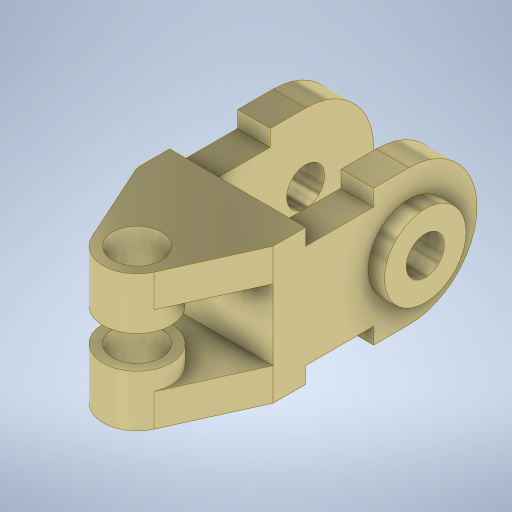
# Autodesk Inventor part: Opakování_1
Saved by Autodesk Inventor 2023 (Build 270158000, 158)
## iProperties
Created: 2023-11-21
Part Number: Opakování_1
Material: Stříbro
Document SubType Name: Modeling
Designer: bit40248
Density: 10.49 g/cm^3
Appearance: Zlato – kov
Mass: 1272.72 g
Surface Area: 310.869 cm^2
Volume: 121.327 cm^3
Author: bit40248
Autodesk Inventor part; units mm, degrees
ref_plane "YZ Plane" through (0, 0, 0) normal (1, 0, 0) x (0, 1, 0)
ref_plane "XZ Plane" through (0, 0, 0) normal (0, 1, 0) x (-1, 0, 0)
ref_plane "XY Plane" through (0, 0, 0) normal (0, 0, 1) x (1, 0, 0)
sketch "Náčrt1" plane through (0, 0, 0) normal (0, 0, 1) x (1, 0, 0)
  line L0 (0, 0) -> (50, 0)
  line L1 (50, 0) -> (50, -50)
  line L2 (50, -50) -> (0, -50)
  line L3 (0, -50) -> (0, 0)
  dimension "d0" = 50
  dimension "d1" = 50
  constraints: 8 end point, 2 parallel, 1 horizontal, 1 perpendicular
  measures "d0" distance of L1.end L2.end
  measures "d1" distance of L0.end L1.end
extrude "Vysunutí1" add sketch "Náčrt1" against normal blind 50
sketch "Náčrt2" plane through (0, 0, 0) normal (0, 1, 0) x (1, 0, 0)
  line L0 (12, 12) -> (38, 12)
  line L1 (38, 12) -> (38, 50)
  line L2 (38, 50) -> (12, 50)
  line L3 (12, 50) -> (12, 12)
  line L4 (0, 50) -> (50, 50) projected
  line L5 (0, 0) -> (0, 50) projected
  dimension "d4" = 12
  dimension "d5" = 26
  dimension "d6" = 38
  constraints: 8 end point, 2 parallel, 1 collinear, 1 horizontal, 1 perpendicular
  measures "d4" distance between parallel lines of L5 L3
  measures "d5" distance between parallel lines of L1 L3
  measures "d6" distance between parallel lines of L0 L2
extrude "Vysunutí2" cut sketch "Náčrt2" against normal blind 50
sketch "Náčrt3" plane through (50, -50, 0) normal (1, 0, 0) x (0, 0, -1)
  line L0 (12, 50) -> (37, 50)
  line L1 (37, 50) -> (37, 44)
  line L2 (37, 44) -> (12, 44)
  line L3 (12, 44) -> (12, 50)
  line L4 (0, 50) -> (50, 50) projected
  line L5 (0, 0) -> (0, 50) projected
  point P0 (37, 47)
  point P1 (12, 47)
  dimension "d9" = 12
  dimension "d10" = 25
  dimension "d11" = 6
  constraints: 8 end point, 2 midpoint, 2 parallel, 1 collinear, 1 horizontal, 1 perpendicular
  measures "d9" distance between parallel lines of L5 L3
  measures "d10" distance of point (37, 47) point (12, 47)
  measures "d11" distance between parallel lines of L2 L4
extrude "Vysunutí3" cut sketch "Náčrt3" against normal blind 50
sketch "Náčrt4" plane through (50, -50, 0) normal (1, 0, 0) x (0, 0, -1)
  line L0 (12, 6) -> (37, 6)
  line L1 (37, 6) -> (37, 0)
  line L2 (37, 0) -> (12, 0)
  line L3 (12, 0) -> (12, 6)
  line L4 (0, 0) -> (50, 0) projected
  line L5 (0, 0) -> (0, 50) projected
  point P0 (37, 3)
  point P1 (12, 3)
  dimension "d14" = 12
  dimension "d15" = 6
  dimension "d16" = 25
  constraints: 8 end point, 2 midpoint, 2 parallel, 1 collinear, 1 horizontal, 1 perpendicular
  measures "d14" distance between parallel lines of L5 L3
  measures "d15" distance between parallel lines of L2 L0
  measures "d16" distance of point (37, 3) point (12, 3)
extrude "Vysunutí4" cut sketch "Náčrt4" against normal blind 50
sketch "Náčrt5" plane through (50, -50, 0) normal (1, 0, 0) x (0, 0, -1)
  line L0 (50, 0) -> (50, 50) projected
  arc A0 (50, 0) -> (50, 50) centre (50, 25) ccw
  point P0 (0, 50)
  constraints: 2 end point, 2 point on circle, 1 centre point, 1 midpoint
extrude "Vysunutí5" add sketch "Náčrt5" against normal blind 50
sketch "Náčrt6" plane through (38, 0, -37) normal (0, 1, 0) x (1, 0, 0)
  line L0 (-26, 13) -> (-38, 13) projected
  line L1 (-26, 13) -> (0, 13)
  line L2 (0, 13) -> (0, 55.1409)
  line L3 (0, 55.1409) -> (-26, 55.1409)
  line L4 (-26, 55.1409) -> (-26, 13)
  point P0 (-38, -37)
  constraints: 8 end point, 2 parallel, 1 horizontal, 1 perpendicular
extrude "Vysunutí6" cut sketch "Náčrt6" against normal blind 50
sketch "Náčrt7" plane through (50, -50, 0) normal (1, 0, 0) x (0, 0, -1)
  circle A0 centre (50, 25) radius 15
  point P0 (0, 50)
  dimension "d23" = 30
  constraints: 1 centre point
  measures "d23" diameter of A0
extrude "Vysunutí7" add sketch "Náčrt7" along normal blind 6
sketch "Náčrt8" plane through (0, -50, 0) normal (-1, 0, 0) x (0, 0, 1)
  circle A0 centre (-50, 25) radius 15 projected
  circle A1 centre (-50, 25) radius 15
  point P0 (0, 50)
  constraints: 1 centre point, 1 coincident
extrude "Vysunutí8" add sketch "Náčrt8" along normal blind 6
sketch "Náčrt9" plane through (-6, -25, -50) normal (-1, 0, 0) x (0, 0, 1)
  circle A0 centre (0, 0) radius 7
  point P0 (50, 25)
  dimension "d28" = 14
  constraints: 1 centre point
  measures "d28" diameter of A0
extrude "Vysunutí9" cut sketch "Náčrt9" against normal blind 100
sketch "Náčrt10" plane through (0, 0, 0) normal (0, 1, 0) x (1, 0, 0)
  circle A0 centre (25, -25) radius 12.5
  line L0 (0, 0) -> (13.607, -30.143)
  line L1 (50, 0) -> (50, 12) projected
  line L2 (50, 0) -> (36.393, -30.143)
  dimension "d31" = 25
  constraints: 4 end point, 2 point on circle, 2 tangent, 1 centre point, 1 other
  measures "d31" diameter of A0
extrude "Vysunutí10" add sketch "Náčrt10" against normal blind 50
sketch "Náčrt11" plane through (25, 0, 25) normal (0, 1, 0) x (1, 0, 0)
  point P0 (-25, 25)
sketch "Náčrt12" plane through (0, 0, 0) normal (0, 1, 0) x (1, 0, 0)
  line L0 (50, 0) -> (0, 0) projected
  line L1 (0, 0) -> (13.607, -30.143)
  line L2 (50, 0) -> (36.393, -30.143)
  circle A0 centre (25, -25) radius 12.5 projected
  constraints: 4 end point, 2 point on circle, 2 tangent
extrude "Vysunutí11" add sketch "Náčrt12" against normal blind 12 contours L2 A0 L1 L0
sketch "Náčrt13" plane through (0, -50, 0) normal (0, -1, 0) x (1, 0, 0)
  line L0 (50, 0) -> (50, -12) projected
  line L1 (50, 0) -> (36.393, 30.143)
  line L2 (13.607, 30.143) -> (0, 0) projected
  line L3 (0, 0) -> (13.607, 30.143)
  circle A0 centre (25, 25) radius 12.5 projected
  line L4 (50, 0) -> (50, -12) projected
  line L5 (0, 0) -> (0, -12) projected
  line L6 (50, 0) -> (0, 0)
  constraints: 6 end point, 2 point on circle, 2 tangent
extrude "Vysunutí12" add sketch "Náčrt13" against normal blind 12 contours L6 L2 A0 L1
sketch "Náčrt16" plane through (0, 0, 0) normal (0, 0, 1) x (1, 0, 0)
  point P0 (0, 0)
sketch "Náčrt17" plane through (0, 0, 0) normal (0, 0, 1) x (1, 0, 0)
  point P0 (0, 0)
sketch "Náčrt18" plane through (0, 0, 0) normal (0, 0, 1) x (1, 0, 0)
  line L0 (50, -10) -> (50, -40) projected
  line L1 (0, 0) -> (0, -50) projected
  line L2 (50, -19) -> (0, -19)
  line L3 (0, -19) -> (0, -31)
  line L4 (0, -31) -> (50, -31)
  line L5 (50, -31) -> (50, -19)
  dimension "d38" = 12
  constraints: 8 end point, 2 parallel, 2 point on line, 1 horizontal, 1 perpendicular
  measures "d38" distance of L3.end L2.end
extrude "Vysunutí13" cut sketch "Náčrt18" along normal blind 100
sketch "Náčrt19" plane through (0, -50, -12) normal (0, -1, 0) x (1, 0, 0)
  arc A0 (13.607, 42.143) -> (36.393, 42.143) centre (25, 37) ccw projected
  circle A1 centre (25, 37) radius 9
  point P0 (0, 12)
  dimension "d41" = 18
  constraints: 1 centre point, 1 coincident
  measures "d41" diameter of A1
extrude "Vysunutí14" cut sketch "Náčrt19" against normal blind 100
